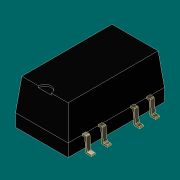
# Autodesk Inventor part: PDS1-M
Saved by Autodesk Inventor 2016 SP1 (Build 200210100, 210)
## iProperties
Created: 2016-04-06
Part Number: PDS1-M
Material: ABS Plastic
Document SubType Name: Modeling
Designer: sawai
Density: 1.06 g/cm^3
Appearance: Smooth - Black
Author: sawai
Autodesk Inventor part; units mm, degrees
ref_plane "YZ Plane" through (0, 0, 0) normal (1, 0, 0) x (0, 1, 0)
ref_plane "XZ Plane" through (0, 0, 0) normal (0, 1, 0) x (-1, 0, 0)
sketch "Sketch1" plane through (0, 0, 0) normal (0, 1, 0) x (-1, 0, 0)
  line L0 (-4.15, 7.62) -> (4.15, 7.62)
  line L1 (4.15, 7.62) -> (4.15, -7.62)
  line L2 (4.15, -7.62) -> (-4.15, -7.62)
  line L3 (-4.15, -7.62) -> (-4.15, 7.62)
  line L4 (-4.15, 7.62) -> (4.15, -7.62) construction
  line L5 (4.15, 7.62) -> (-4.15, -7.62) construction
  point P0 (0, 0)
  dimension "d0" = 8.3
  dimension "d1" = 15.24
  constraints: 12 end point, 2 midpoint, 2 parallel, 1 horizontal, 1 perpendicular
  measures "d0" distance of L1.end L2.end
  measures "d1" distance of L0.end L1.end
extrude "Extrusion1" add sketch "Sketch1" along normal blind 7
chamfer "Chamfer1" distance 0.5 distance2 5 1 edges at (4.15, 7, 0) measured on face at (3.65, 7, 0)
chamfer "Chamfer2" distance 0.5 distance2 5 1 edges at (-4.15, 7, 0) measured on face at (-3.65, 7, 0)
chamfer "Chamfer3" distance 0.5 distance2 5 1 edges at (0, 7, 7.62) measured on face at (0, 7, 7.12)
chamfer "Chamfer4" distance 0.5 distance2 5 1 edges at (0, 7, -7.62) measured on face at (0, 7, -7.12)
sketch "Sketch2" plane through (0, 7, 0) normal (0, 1, 0) x (1, 0, 0)
  line L0 (-3.65, 7.12) -> (3.65, 7.12) projected
  line L1 (-3.65, -7.12) -> (-3.65, 7.12) projected
  line L2 (3.65, -7.12) -> (-3.65, -7.12) projected
  line L3 (3.65, 7.12) -> (3.65, -7.12) projected
  line L4 (3.65, -7.12) -> (-3.65, -7.12) projected
  circle A0 centre (0, -7.12) radius 1
  point P0 (0, 0)
  dimension "d16" = 2
  constraints: 1 centre point, 1 midpoint
  measures "d16" diameter of A0
extrude "Extrusion2" cut sketch "Sketch2" against normal blind 0.25 contours A0 L2 | L2 A0
ref_plane "Work Plane1" through (0, 0, 5.08) normal (0, 0, 1) x (1, 0, 0)
sketch "Sketch3" plane through (0, 0, 5.08) normal (0, 0, 1) x (1, 0, 0)
  line L0 (-4.15, 2) -> (4.15, 2) projected
  line L1 (-4.15, 0) -> (-4.15, 2) projected
  line L2 (4.15, 0) -> (-4.15, 0) projected
  line L3 (4.15, 0) -> (4.15, 2) projected
  ellipse E0 centre (0, 7) end of major axis (0, 17) minor radius 1 (0.9997, 6.75) -> (1, 7) ccw projected
  line L4 (0.9997, 6.75) -> (-0.9997, 6.75) projected
  ellipse E1 centre (0, 7) end of major axis (0, 17) minor radius 1 (-1, 7) -> (-0.9997, 6.75) ccw projected
  line L5 (-1, 7) -> (-3.65, 7) projected
  line L6 (-3.65, 7) -> (-4.15, 2) projected
  line L7 (-4.15, 2) -> (4.15, 2) projected
  line L8 (4.15, 2) -> (3.65, 7) projected
  line L9 (3.65, 7) -> (1, 7) projected
  line L10 (4.15, 1.875) -> (4.5341, 1.875)
  line L11 (4.5341, 1.875) -> (4.72, -0.25)
  line L12 (4.72, -0.25) -> (5.6, -0.25)
  line L13 (5.6, -0.25) -> (5.6, 0)
  line L14 (5.6, 0) -> (4.9491, 0)
  line L15 (4.9491, 0) -> (4.7632, 2.125)
  line L16 (4.7632, 2.125) -> (4.1375, 2.125)
  line L17 (4.15, 2) -> (3.65, 7) projected
  line L18 (4.1375, 2.125) -> (4.15, 2)
  line L19 (4.15, 2) -> (4.15, 1.875)
  line L20 (4.15, 0) -> (4.15, 2) projected
  point P0 (0, 0)
  dimension "d20" = 0.25
  dimension "d21" = 0.125
  dimension "d22" = 0.25
  dimension "d23" = 0.25
  dimension "d24" = 0.25
  dimension "d25" = 0.57
  dimension "d26" = 1.45
  dimension "d27" = 95
  constraints: 18 end point, 3 parallel, 2 collinear, 2 perpendicular, 2 point on line, 1 horizontal, 2 other
  measures "d20" distance between parallel lines of L16 L10
  measures "d21" distance between parallel lines of L0 L10
  measures "d22" distance between parallel lines of L15 L11
  measures "d23" distance between parallel lines of L2 L12
  measures "d24" distance between parallel lines of L12 L14
  measures "d25" distance from line of L3 L11.end
  measures "d26" distance from line of L3 L12.end
  measures "d27" angle of L10 L11
extrude "Extrusion3" add sketch "Sketch3" along normal mid plane 0.6 separate body contours L8 L16 L15 L14 L13 L12 L11 L10 L3
fillet "Fillet1" radius 0.1 5 edges at (4.7632, 2.125, 5.08) (4.5341, 1.875, 5.08) (4.9491, 0, 5.08) (4.72, -0.25, 5.08) (5.6, 0, 5.08)
pattern_linear "Rectangular Pattern1" count 5 spacing 2.54 along (0, 0, -1) of "Extrusion3", "Fillet1" bodies 2
mirror "Mirror1" about plane through (0, 0, 0) normal (1, 0, 0) of "Extrusion3", "Rectangular Pattern1", "Fillet1" bodies 2
sketch "Sketch4" plane through (4.72, -0.25, 0.3) normal (0, -1, 0) x (1, 0, 0)
  line L0 (3.3959, -1.0729) -> (-2.0663, -1.0729)
  line L1 (-2.0663, -1.0729) -> (-2.0663, 0.5586)
  line L2 (-2.0663, 0.5586) -> (3.3959, 0.5586)
  line L3 (3.3959, 0.5586) -> (3.3959, -1.0729)
  line L4 (-11.2171, -4.2651) -> (-6.3934, -4.2651)
  line L5 (-6.3934, -4.2651) -> (-6.3934, -6.7479)
  line L6 (-6.3934, -6.7479) -> (-11.2171, -6.7479)
  line L7 (-11.2171, -6.7479) -> (-11.2171, -4.2651)
  line L8 (-13.0615, 3.538) -> (-5.8968, 3.538)
  line L9 (-5.8968, 3.538) -> (-5.8968, -1.5695)
  line L10 (-5.8968, -1.5695) -> (-13.0615, -1.5695)
  line L11 (-13.0615, -1.5695) -> (-13.0615, 3.538)
  constraints: 24 end point, 6 parallel, 3 horizontal, 3 perpendicular
extrude "Extrusion4" cut sketch "Sketch4" along normal through all both and the other way through all bodies 2
body "Solid1"
body "Solid2"
